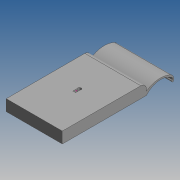
# Autodesk Inventor part: P052_BasGrenouillere
Saved by Autodesk Inventor 2021.3 (Build 253353000, 353)
## iProperties
Created: 2022-01-14
Part Number: P052_BasGrenouillere
Material: Générique
Document SubType Name: Modeling
Designer: gabri
Density: 1 g/cm^3
Appearance: Par défaut
Author: gabri
Autodesk Inventor part; units mm, degrees
ref_plane "YZ Plane" through (0, 0, 0) normal (1, 0, 0) x (0, 1, 0)
ref_plane "XZ Plane" through (0, 0, 0) normal (0, 1, 0) x (-1, 0, 0)
ref_plane "XY Plane" through (0, 0, 0) normal (0, 0, 1) x (1, 0, 0)
sketch "Sketch2" plane through (0, 0, 0) normal (0, 0, 1) x (1, 0, 0)
  line L0 (10, -15) -> (-10, -15)
  line L1 (-10, -15) -> (-10, 15)
  line L2 (-10, 15) -> (10, 15)
  line L3 (10, 15) -> (10, -15)
  line L4 (10, -15) -> (-10, 15) construction
  line L5 (-10, -15) -> (10, 15) construction
  circle A0 centre (0, 1.0833) radius 0.6009
  line L6 (0.5, 0.75) -> (-0.5, 0.75)
  line L7 (-0.5, 0.75) -> (-0.5, -0.75)
  line L8 (-0.5, -0.75) -> (0.5, -0.75)
  line L9 (0.5, -0.75) -> (0.5, 0.75)
  line L10 (0, 21) -> (0, -21) construction
  point P0 (0, 0)
  point P1 (-0.5, 0.75)
  dimension "d0" = 20
  dimension "d1" = 30
  dimension "d4" = 0.5
  dimension "d5" = 0.5
  constraints: 20 end point, 4 parallel, 3 point on line, 2 horizontal, 2 midpoint, 2 perpendicular, 4 other
  measures "d0" distance of L1.end L2.end
  measures "d1" distance between parallel lines of L0 L2
  measures "d4" distance between parallel lines of L10 L9
  measures "d5" distance between parallel lines of L10 L7
extrude "Extrusion1" add sketch "Sketch2" along normal blind 4
sketch "Sketch3" plane through (0, 0, 4) normal (0, 0, 1) x (1, 0, 0)
  point P0 (0, 0)
sketch "Sketch4" plane through (-10, -15, 0) normal (-1, 0, 0) x (0, 0, 1)
  line L0 (0, 30) -> (0, 0) construction
  line L1 (0, 0) -> (4, 0) construction
  line L2 (4, 30) -> (4, 0) construction
  line L3 (0, 30) -> (4, 30) construction
  line L4 (0, 46.4166) -> (0, -7.7361) construction
  arc A0 (1.298, 30) -> (1.9002, 38.9656) centre (-5.508, 34.9602) ccw
  arc A1 (0, 30) -> (0.9317, 39.23) centre (-4.2199, 35.088) ccw
  arc A2 (0.9317, 39.23) -> (0.1696, 39.2983) centre (0.4574, 38.2233) ccw
  arc A3 (1.9002, 38.9656) -> (-0.2384, 39.6889) centre (0.2326, 37.5581) ccw
  arc A4 (-0.2384, 39.6889) -> (0.1696, 39.2983) centre (-0.1651, 39.3571) ccw
  line L5 (0, 30) -> (4, 30) construction
  line L6 (0, 30) -> (1.298, 30)
  point P0 (0, 15)
  point P1 (0, 37.5)
  dimension "d74" = 1.1128
  dimension "d75" = 2.1822
  dimension "d76" = 0.3398
  dimension "d77" = 6.6102
  dimension "d78" = 8.4217
  dimension "d79" = 2.0998
  dimension "d80" = 8.9656
  dimension "d81" = 2.702
  dimension "d82" = 3.0683
  dimension "d83" = 9.23
  dimension "d84" = 3.5426
  dimension "d85" = 3.7674
  dimension "d86" = 3.8304
  dimension "d87" = 7.5
  constraints: 10 point on circle, 5 centre point, 2 end point, 2 point on line, 1 collinear, 1 tangent, 1 vertical, 2 other
  measures "d74" radius of A2
  measures "d75" radius of A3
  measures "d76" radius of A4
  measures "d77" radius of A1
  measures "d78" radius of A0
  measures "d79" distance from line of A0.end L2
  measures "d80" distance from line of A0.end L5
  measures "d81" distance from line of L6.end L2
  measures "d82" distance from line of A1.end L2
  measures "d83" distance from line of A1.end L5
  measures "d84" distance from line of A2.centre L2
  measures "d85" distance from line of A3.centre L2
  measures "d86" distance from line of A2.end L2
  measures "d87" distance from line of point (0, 37.5) L5
extrude "Extrusion2" add sketch "Sketch4" against normal up to surface (20 mm away)
fillet "Fillet1" radius 2 1 edges at (0, 23.9656, 1.9002)
fillet "Fillet2" radius 2 1 edges at (0, 15, 4)
body "Solid1"
